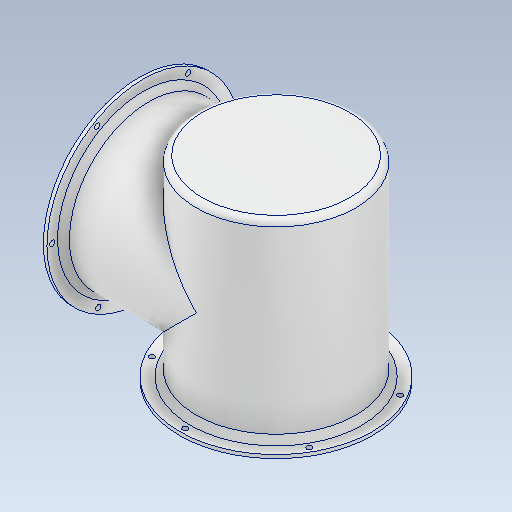
# Autodesk Inventor part: Link_2_b
Saved by Autodesk Inventor 2021 (Build 250183000, 183)
## iProperties
Created: 2020-05-10
Part Number: Link_2_b
Material: Aluminum 6061
Document SubType Name: Modeling
Designer: avi41
Density: 2.7 g/cm^3
Appearance: Aluminum - Flat
Mass: 384.639 g
Surface Area: 3507.09 cm^2
Volume: 384.639 cm^3
Author: avi41
Autodesk Inventor part; units mm, degrees
note: some values were not read from the file. Chosen so that the rebuilt part matches the saved one: direction of "Hole2".
ref_plane "XZ Plane" through (0, 0, 0) normal (0, 1, 0) x (-1, 0, 0)
sketch "Sketch1" plane through (0, 0, 0) normal (0, 0, 1) x (1, 0, 0)
  line L0 (-16.3, 0) -> (97.8, 0) construction
  line L1 (0, 163.5) -> (0, -123.5) construction
  line L2 (65.5, -82.5) -> (65.5, 79.5)
  line L3 (81.5, -79.5) -> (81.5, -82.5)
  line L4 (81.5, -82.5) -> (65.5, -82.5)
  line L5 (67.5, -74.5) -> (67.5, 82.5)
  line L6 (81.5, -79.5) -> (72.5, -79.5)
  line L7 (72.5, -79.5) -> (67.5, -74.5)
  line L8 (67.5, 82.5) -> (0, 82.5)
  line L9 (0, 122.5) -> (0, 120.5)
  line L10 (0, 79.5) -> (0, 82.5)
  line L11 (0, 79.5) -> (65.5, 79.5)
  point P0 (0, 0)
  dimension "d5" = 81.5
  dimension "d7" = 9
  dimension "d8" = 5
  dimension "d9" = 45
  dimension "d10" = 16
  dimension "d11" = 3
  dimension "d32" = 2
  dimension "d34" = 165
  dimension "d125" = 3
  constraints: 20 end point, 4 point on line, 3 perpendicular, 2 collinear, 1 horizontal, 1 vertical, 1 other
  measures "d5" distance between parallel lines of L1 L3
  measures "d7" distance of L3.start L6.end
  measures "d8" horizontal distance of L6.end L5.start
  measures "d9" angle of L4 L7
  measures "d10" distance of L3.end L2.start
  measures "d11" distance between parallel lines of L4 L6
  measures "d32" distance between parallel lines of L5 L2
  measures "d34" distance between parallel lines of L4 L8
  measures "d125" distance between parallel lines of L11 L8
revolve "Revolution1" add sketch "Sketch1" angle 360 about axis through (0, 0, 0) along (0, -1, 0)
sketch "Sketch2" plane through (0, -82.5, 0) normal (0, -1, 0) x (1, 0, 0)
  line L0 (0, 114.1) -> (0, -114.1) construction
  line L1 (-114.1, 0) -> (114.1, 0) construction
  circle A0 centre (0, 0) radius 81.5 construction
  circle A1 centre (0, 0) radius 65.5 construction
  circle A2 centre (0, 0) radius 77 construction
  circle A3 centre (0, 0) radius 72.5 construction
  point P0 (0, 77)
  point P1 (-66.684, 38.5)
  point P2 (-66.684, -38.5)
  point P3 (0, -77)
  point P4 (66.684, -38.5)
  point P5 (66.684, 38.5)
  dimension "d16" = 4.5
  dimension "d20" = 360
  dimension "d29" = 4.5
  constraints: 1 coincident, 1 point on line, 1 vertical alignment, 9 other
hole "Hole1" at (0, -82.5, 77) at (-66.684, -82.5, 38.5) at (-66.684, -82.5, -38.5) at (0, -82.5, -77) at (66.684, -82.5, -38.5) at (66.684, -82.5, 38.5) direction (0, 1, 0) diameter 4.5 depth 13 tip angle 118 clearance for "Flat Head Machine Screw" size "M4" standard "Ansi Metric M Profile"
fillet "Fillet1" radius 5 1 edges at (-67.5, 82.5, 0)
ref_plane "Work Plane1" through (-67.5, 4, 0) normal (1, 0, 0) x (0, 1, 0)
sketch "Sketch6" plane through (-67.5, 4, 0) normal (1, 0, 0) x (0, 1, 0)
  line L0 (-78.5, 67.5) -> (-78.5, -67.5) construction
  line L1 (-3.5, 87.6289) -> (-3.5, -132.6334) construction
  circle A0 centre (-3.5, 0) radius 67.5
  line L2 (-134, 0) -> (198.5, 0) construction
  point P0 (-4, 0)
  point P1 (151, -67.5)
  point P2 (151, 67.5)
  dimension "d50" = 135
  dimension "d92" = 75
  constraints: 2 end point, 2 point on line, 1 centre point, 1 vertical
  measures "d50" diameter of A0
  measures "d92" distance between parallel lines of L0 L1
extrude "Extrusion3" add sketch "Sketch6" along normal up to surface (67.5 mm away)
extrude "Extrusion5" add sketch "Sketch6" against normal blind 48
sketch "Sketch7" plane through (0, 0, 0) normal (1, 0, 0) x (0, 1, 0)
  line L0 (16.8095, -65.5) -> (-15.8095, -65.5) projected
  line L1 (-15.8095, 65.5) -> (16.8095, 65.5) projected
  arc A0 (-15.8095, 65.5) -> (-15.8095, -65.5) centre (0.5, 0) ccw projected
  arc A1 (16.8095, -65.5) -> (16.8095, 65.5) centre (0.5, 0) ccw projected
  arc A2 (16.3263, -63.5593) -> (16.5624, 63.5) centre (0.5, 0) ccw
  line L2 (16.5624, 63.5) -> (-15.5624, 63.5)
  arc A3 (-15.5624, 63.5) -> (-15.5624, -63.5) centre (0.5, 0) ccw
  line L3 (-15.5624, -63.5) -> (17.8095, -63.5)
  point P0 (16.5624, -63.5)
  dimension "d74" = 2
  constraints: 4 end point, 4 point on circle, 2 centre point, 3 other
  measures "d74" radial gap between concentric circles of A0 A3
extrude "Extrusion4" cut sketch "Sketch7" against normal blind 112 contours L3 A3 L2 A2
sketch "Sketch5" plane through (0, 0, 0) normal (0, 0, 1) x (1, 0, 0)
  line L0 (-112.5, -81) -> (-112.5, -72)
  line L1 (-115.5, -67) -> (-67.5, -67) construction
  line L2 (-115.5, 68) -> (-115.5, -67) construction
  line L3 (-115.5, 68) -> (-67.5, 68) construction
  line L4 (-36.372, 0.5) -> (-151.0487, 0.5) construction
  line L5 (-107.5, -67) -> (-112.5, -72)
  line L6 (-112.5, -81) -> (-115.5, -81)
  line L7 (-115.5, -81) -> (-115.5, -67)
  line L8 (-107.5, -67) -> (-115.5, -67)
  point P0 (0, 0)
  point P1 (0, 0)
  point P2 (0, 0)
  point P3 (0, 0)
  point P4 (0, 0)
  dimension "d43" = 9
  dimension "d59" = 67.5
  dimension "d62" = 5
  dimension "d63" = 45
  dimension "d75" = 3
  dimension "d76" = 67.5
  constraints: 12 end point, 2 coincident, 2 horizontal, 1 collinear, 1 perpendicular, 1 vertical
  measures "d43" distance of L0.start L0.end
  measures "d59" distance between parallel lines of L3 L4
  measures "d62" horizontal distance of L5.start L0.end
  measures "d63" angle of L0 L5
  measures "d75" distance of L0.start L6.end
  measures "d76" distance between parallel lines of L4 L1
revolve "Revolution2" add sketch "Sketch5" angle 360 about axis through (-36.372, 0.5, 0) along (-1, 0, 0)
sketch "Sketch8" plane through (-115.5, 0.5, 0) normal (-1, 0, 0) x (0, 0, 1)
  circle A0 centre (0, 0) radius 65.5
  circle A1 centre (0, 0) radius 81.5 projected
  circle A2 centre (0, 0) radius 67.5 projected
  point P0 (0, -0.5)
  dimension "d78" = 2
  constraints: 1 centre point, 1 coincident
  measures "d78" radial gap between concentric circles of A0 A2
extrude "Extrusion6" cut sketch "Sketch8" against normal up to surface (115.5 mm away) contours A0
sketch "Sketch11" plane through (-115.5, 0.5, 0) normal (-1, 0, 0) x (0, 0, 1)
  circle A0 centre (0, 0) radius 81.5 construction
  circle A1 centre (0, 0) radius 65.5 construction
  line L0 (-114.1, -0.5) -> (114.1, -0.5) construction
  line L1 (0, 115) -> (0, -116) construction
  circle A2 centre (0, 0) radius 72.5 projected
  circle A3 centre (0, 0) radius 77 construction
  point P0 (0, -0.5)
  point P1 (76.9984, -0.5)
  point P2 (38.9322, 66.4326)
  point P3 (-38.0662, 66.9326)
  point P4 (-76.9984, 0.5)
  point P5 (-38.9322, -66.4326)
  point P6 (38.0662, -66.9326)
  dimension "d79" = 4.5
  dimension "d80" = 4.5
  dimension "d83" = 360
  constraints: 1 coincident, 1 point on line, 10 other
hole "Hole2" at (-115.5, 0, 76.9984) at (-115.5, 66.9326, 38.9322) at (-115.5, 67.4326, -38.0662) at (-115.5, 1, -76.9984) at (-115.5, -65.9326, -38.9322) at (-115.5, -66.4326, 38.0662) direction (1, 0, 0) diameter 4.5 depth 3 clearance for "Flat Head Machine Screw" size "M4" standard "Ansi Metric M Profile"
sketch "Sketch9" plane through (0, -82.5, 0) normal (0, -1, 0) x (1, 0, 0)
  circle A0 centre (0, 0) radius 65.5 projected
  dimension "d93" = 135
  dimension "d95" = 72
extrude "Extrusion7" cut sketch "Sketch9" against normal up to surface (162 mm away)
ref_plane "Work Plane2" through (0, 4, 67.5) normal (0, 0, 1) x (1, 0, 0)
sketch "Sketch14" plane through (0, 50.5, 102.5) normal (0, 0, 1) x (1, 0, 0)
  circle A0 centre (0, 0) radius 67.5 construction
  circle A1 centre (0, 0) radius 65.5
  point P0 (0, -50.5)
  dimension "d100" = 2
  constraints: 1 centre point
  measures "d100" radial gap between concentric circles of A0 A1
sketch "Sketch15" plane through (0, 0, 0) normal (1, 0, 0) x (0, 1, 0)
  line L0 (-31, 99.5) -> (-22, 99.5)
  line L1 (-17, 94.5) -> (-22, 99.5)
  line L2 (-31, 99.5) -> (-31, 102.5)
  line L3 (-31, 102.5) -> (-17, 102.5)
  line L4 (-17, 94.5) -> (-17, 102.5)
  line L5 (118, 102.5) -> (118, 67.4749) construction
  line L6 (-15, 102.5) -> (116, 102.5) construction
  line L7 (118, 102.5) -> (-17, 102.5) construction
  line L8 (-17, 102.5) -> (-17, 67.5) construction
  line L9 (-17, 102.5) -> (-17, 67.5) construction
  line L10 (50.5, 133.3679) -> (50.5, 80.094) construction
  point P0 (0, 0)
  point P1 (0, 0)
  point P2 (0, -80)
  point P3 (0, -80)
  point P4 (0, 69)
  point P5 (0, 69)
  dimension "d103" = 9
  dimension "d105" = 5
  dimension "d106" = 45
  dimension "d107" = 3
  dimension "d109" = 67.5
  dimension "d110" = 67.5
  constraints: 12 end point, 2 coincident, 2 collinear, 2 parallel, 1 perpendicular, 1 vertical, 4 other
  measures "d103" distance of L0.start L0.end
  measures "d105" horizontal distance of L1.start L0.end
  measures "d106" angle of L0 L1
  measures "d107" distance of L0.start L2.end
  measures "d109" distance between parallel lines of L10 L5
  measures "d110" distance between parallel lines of L8 L10
sketch "Sketch16" plane through (0, 50.5, 102.5) normal (0, 0, 1) x (1, 0, 0)
  circle A0 centre (0, 0) radius 72.5 construction
  circle A1 centre (0, 0) radius 81.5 construction
  line L0 (0, 0) -> (126.1928, 0) construction
  line L1 (0, 132.4) -> (0, -223.9) construction
  circle A2 centre (0, 0) radius 77 construction
  point P0 (0, -50.5)
  point P1 (77, 0)
  point P2 (38.5, -66.684)
  point P3 (-38.5, -66.684)
  point P4 (-77, 0)
  point P5 (-38.5, 66.684)
  point P6 (38.5, 66.684)
  dimension "d112" = 4.5
  dimension "d113" = 4.5
  dimension "d116" = 360
  constraints: 2 end point, 1 coincident, 1 horizontal, 1 horizontal alignment, 1 point on line, 9 other
equation "\"d16\" = d29"
equation "\"d76\" = d59"
equation "\"d79\" = d80"
body "Solid1"
